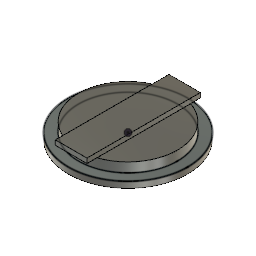
big flapper plate v3 (Autodesk Fusion 360 design; units mm, degrees)
Autodesk Fusion 360 part; units mm, degrees
sketch "Sketch1" plane through (0, 0, 0) normal (0, 0, 1) x (1, 0, 0)
  circle A0 centre (0, 0) radius 15.65
  circle A1 centre (0, 0) radius 18.9
  dimension "d3" = 31.3
  dimension "d11" = 37.8
  constraint coincident A0.centre A1.centre
  measures "d3" diameter of A0
  measures "d11" diameter of A1
extrude "Extrude1" add sketch "Sketch1" along normal blind 3 contours A0
sketch "Sketch2" plane through (0, 0, 3) normal (0, 0, 1) x (-1, 0, 0)
  circle A0 centre (0, 0) radius 15.65
  line L0 (-5, -18) -> (5, -18)
  line L1 (5, -18) -> (5, 18)
  line L2 (5, 18) -> (-5, 18)
  line L3 (-5, 18) -> (-5, -18)
  line L4 (-5, -18) -> (5, 18) construction
  line L5 (5, -18) -> (-5, 18) construction
  dimension "d7" = 10
  dimension "d8" = 36
  constraint horizontal L0
  constraint perpendicular L0 L1
  constraint parallel L0 L2
  constraint parallel L1 L3
  constraint coincident L4 A0.centre
  constraint coincident L5 A0.centre
  constraint coincident A0.centre origin
  measures "d7" distance of L1.end L2.end
  measures "d8" distance of L0.end L1.end
extrude "Extrude2" add sketch "Sketch2" along normal blind 1.5 contours A0 L1 L3 | A0 L1 L2 L3 | A0 L0 L1 L3
extrude "Extrude3" add sketch "Sketch1" against normal blind 2 contours A0 | A1
equation "bigID = 31.3 mm"
equation "bigtab = 36 mm"
equation "d3 = bigID"
equation "bigtabwidth = 10 mm"
equation "d7 = bigtabwidth"
equation "d8 = bigtab"
equation "d11 = bigID + 6.5 mm"
named bodies: "big flapper"
